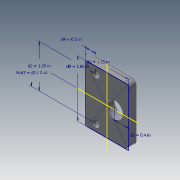
# Autodesk Inventor part: Standard
Saved by Autodesk Inventor 2020.3 (Build 243373000, 373)
## iProperties
RuleStatus: InUse
AfterDocSave0: file://Part Number Cleaner
Created: 2023-02-07
Material: Generic
Catalog Web Link: https://www.janelia.org/
Vendor: HHMI: JRC - jET
Document SubType Name: Modeling
Designer: arnoldj
Density: 1 g/cm^3
Appearance: Default
DESIGN DEPARTMENT: HHMI: JRC - jET
ALTERED ITEM PART NUMBER: N/A
ALTERED ITEM VENDOR: N/A
ALTERED ITEM DESCRIPTION: N/A
Title: Standard
Author: arnoldj
Revision Number: 0
Autodesk Inventor part; units mm, degrees
ref_plane "YZ Plane" through (0, 0, 0) normal (1, 0, 0) x (0, 1, 0)
ref_plane "XZ Plane" through (0, 0, 0) normal (0, 1, 0) x (-1, 0, 0)
ref_plane "XY Plane" through (0, 0, 0) normal (0, 0, 1) x (1, 0, 0)
sketch "Sketch1" plane through (0, 0, 0) normal (0, 0, 1) x (1, 0, 0)
  line L0 (0, 29.337) -> (0, -29.337) projected
  line L1 (-22.225, 0) -> (22.225, 0) projected
  line L2 (15.875, -20.955) -> (-15.875, -20.955)
  line L3 (-15.875, -20.955) -> (-15.875, 20.955)
  line L4 (-15.875, 20.955) -> (15.875, 20.955)
  line L5 (15.875, 20.955) -> (15.875, -20.955)
  line L6 (15.875, -20.955) -> (-15.875, 20.955) construction
  line L7 (-15.875, -20.955) -> (15.875, 20.955) construction
  point P0 (0, 0)
  point P1 (-8.255, 15.875)
  point P2 (-8.255, -15.875)
  point P3 (5.715, 0)
  dimension "d0" = 41.91
  dimension "d1" = 31.75
  dimension "d2" = 31.75
  dimension "d3" = 15.875
  dimension "d4" = 7.62
  dimension "d5" = 10.16
  constraints: 12 end point, 2 midpoint, 2 parallel, 1 horizontal, 1 perpendicular, 1 point on line, 1 vertical alignment
  measures "d0" distance of L2.end L3.end
  measures "d1" distance of L3.end L4.end
  measures "d2" distance of point (-8.255, -15.875) point (-8.255, 15.875)
  measures "d3" distance from line of point (-8.255, -15.875) L1
  measures "d4" distance from line of point (-8.255, 15.875) L3
  measures "d5" distance from line of L5 point (5.715, 0)
extrude "Extrusion1" add sketch "Sketch1" against normal blind 5.842
hole "Hole1" at (-8.255, 15.875, 0) at (-8.255, -15.875, 0) direction (0, 0, -1) diameter 5.5118 end through all clearance for "Socket Head Cap Screw" size "M5" standard "Ansi Metric M Profile"
hole "Hole2" at (5.715, 0, 0) direction (0, 0, -1) diameter 12.573 end through all
fillet "Fillet1" radius 3.175 4 edges at (-15.875, -20.955, -2.921) (15.875, -20.955, -2.921) (15.875, 20.955, -2.921) (-15.875, 20.955, -2.921)
equation "\"d3\" = 0.5 * d2"
body "Solid1"
